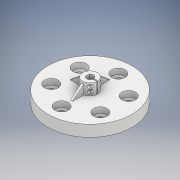
# Autodesk Inventor part: MC001
Saved by Autodesk Inventor 2017 SP1 (Build 210196100, 196)
## iProperties
Created: 2017-06-01
Part Number: MC001
Material: ABS Plastic
Document SubType Name: Modeling
Designer: Zach
Density: 1.06 g/cm^3
Appearance: CR White
Author: Zach
Autodesk Inventor part; units mm, degrees
ref_plane "YZ Plane" through (0, 0, 0) normal (1, 0, 0) x (0, 1, 0)
ref_plane "XY Plane" through (0, 0, 0) normal (0, 0, 1) x (1, 0, 0)
sketch "Sketch1" plane through (0, 0, 0) normal (0, 0, 1) x (1, 0, 0)
  circle A0 centre (0, 0) radius 37
  circle A1 centre (0, 0) radius 3
  circle A2 centre (0, 25) radius 2.575
  circle A3 centre (-21.6506, 12.5) radius 2.575
  circle A4 centre (-21.6506, -12.5) radius 2.575
  circle A5 centre (0, -25) radius 2.575
  circle A6 centre (21.6506, -12.5) radius 2.575
  circle A7 centre (21.6506, 12.5) radius 2.575
  dimension "d0" = 74
  dimension "d1" = 6
  dimension "d2" = 5.15
  dimension "d3" = 25
  dimension "d6" = 360
  constraints: 8 centre point, 2 coincident, 13 other
  measures "d0" diameter of A0
  measures "d1" diameter of A1
  measures "d2" diameter of A2
  measures "d3" distance of point (0, 0) A2.centre
extrude "Extrusion1" add sketch "Sketch1" along normal blind 10
sketch "Sketch2" plane through (0, 0, 10) normal (0, 0, 1) x (1, 0, 0)
  circle A0 centre (0, 0) radius 3 projected
  circle A1 centre (0, 0) radius 6.5
  circle A2 centre (0, 0) radius 3 projected
  dimension "d10" = 13
  constraints: 3 coincident, 1 centre point, 3 other
  measures "d10" diameter of A1
extrude "Extrusion2" add sketch "Sketch2" along normal blind 10
sketch "Sketch3" plane through (0, 0, 10) normal (0, 0, 1) x (1, 0, 0)
  line L0 (0, 0.5) -> (36.9966, 0.5)
  circle A0 centre (0, 0) radius 6.5 projected
  line L1 (0, 0.5) -> (0, -0.5)
  circle A1 centre (0, 0) radius 37 projected
  line L2 (0, -0.5) -> (36.9966, -0.5)
  arc A2 (36.9966, -0.5) -> (36.9966, 0.5) centre (0, 0) ccw
  point P0 (0, 0)
  dimension "d13" = 1
  dimension "d14" = 0.5
  constraints: 6 end point, 4 point on circle, 2 horizontal, 2 vertical alignment, 1 centre point, 1 concentric, 1 midpoint, 1 vertical
  measures "d13" distance of L0.start L1.end
  measures "d14" distance of L0.start point (0, 0)
extrude "Extrusion4" cut sketch "Sketch3" along normal through all contours L0 A0 L2 L1 | L0 A1 L2 A0 picked at (2.1667, 0) picked at (16.6648, -0.2223)
sketch "Sketch4" plane through (0, 0, 0) normal (0, 1, 0) x (-1, 0, 0)
  circle A0 centre (-4.958, 13) radius 1
  circle A1 centre (-4.958, 17) radius 1
  line L0 (-2.958, 10) -> (-6.4807, 10) projected
  line L1 (-6.4807, 20) -> (-2.958, 20) projected
  line L2 (-2.958, 20) -> (-2.958, 10) projected
  point P0 (0, 0)
  dimension "d19" = 2
  dimension "d20" = 2
  dimension "d21" = 3
  dimension "d22" = 3
  dimension "d25" = 2
  dimension "d26" = 2
  constraints: 2 centre point
  measures "d19" diameter of A0
  measures "d20" diameter of A1
  measures "d21" distance from line of A0.centre L0
  measures "d22" distance from line of L1 A1.centre
  measures "d25" distance from line of L2 A0.centre
  measures "d26" distance from line of L2 A1.centre
extrude "Extrusion5" cut sketch "Sketch4" along normal through all both and the other way through all
ref_plane "Work Plane1" through (0, -6.5, 0) normal (0, 1, 0) x (-1, 0, 0)
sketch "Sketch6" plane through (0, -6.5, 0) normal (0, 1, 0) x (-1, 0, 0)
  spline S0 degree 5 poles (-3.958, 13) (-3.958, 13.1746) (-3.9961, 13.3498) (-4.0725, 13.5117) (-4.1803, 13.65) (-4.4348, 13.869) (-4.583, 13.9477) (-4.7351, 13.9925) (-4.882, 14.0068) (-5.1241, 13.9915) (-5.2226, 13.9719) (-5.3158, 13.9412) (-5.403, 13.9006) (-5.5546, 13.8069) (-5.6202, 13.7562) (-5.6812, 13.6984) (-5.7373, 13.6329) (-5.8334, 13.4906) (-5.8743, 13.4151) (-5.9095, 13.3294) (-5.9362, 13.233) (-5.9579, 13.0655) (-5.9613, 13.0002) (-5.9591, 12.9344) (-5.9515, 12.8703) (-5.9066, 12.6381) (-5.84, 12.4944) (-5.7574, 12.3787) (-5.6684, 12.2835) (-5.4331, 12.1055) (-5.2863, 12.0346) (-5.1214, 11.9912) (-4.9425, 11.9823) (-4.6619, 12.04) (-4.5657, 12.0716) (-4.4707, 12.1171) (-4.3797, 12.1768) (-4.1744, 12.3577) (-4.0693, 12.4951) (-3.995, 12.6552) (-3.958, 12.828) (-3.958, 13) knots 0 0 0 0 0 0 0.118573 0.118573 0.118573 0.118573 0.240763 0.240763 0.240763 0.240763 0.331598 0.331598 0.331598 0.331598 0.410987 0.410987 0.410987 0.410987 0.484843 0.484843 0.484843 0.484843 0.529131 0.529131 0.529131 0.529131 0.655639 0.655639 0.655639 0.655639 0.80726 0.80726 0.80726 0.80726 0.884923 0.884923 0.884923 0.884923 1 1 1 1 1 1 projected
  spline S1 degree 5 poles (-3.958, 17) (-3.958, 17.1746) (-3.9961, 17.3498) (-4.0725, 17.5117) (-4.1803, 17.65) (-4.4348, 17.869) (-4.583, 17.9477) (-4.7351, 17.9925) (-4.882, 18.0068) (-5.1241, 17.9915) (-5.2226, 17.9719) (-5.3158, 17.9412) (-5.403, 17.9006) (-5.5546, 17.8069) (-5.6202, 17.7562) (-5.6812, 17.6984) (-5.7373, 17.6329) (-5.8334, 17.4906) (-5.8743, 17.4151) (-5.9095, 17.3294) (-5.9362, 17.233) (-5.9579, 17.0655) (-5.9613, 17.0002) (-5.9591, 16.9344) (-5.9515, 16.8703) (-5.9066, 16.6381) (-5.84, 16.4944) (-5.7574, 16.3787) (-5.6684, 16.2835) (-5.4331, 16.1055) (-5.2863, 16.0346) (-5.1214, 15.9912) (-4.9425, 15.9823) (-4.6619, 16.04) (-4.5657, 16.0716) (-4.4707, 16.1171) (-4.3797, 16.1768) (-4.1744, 16.3577) (-4.0693, 16.4951) (-3.995, 16.6552) (-3.958, 16.828) (-3.958, 17) knots 0 0 0 0 0 0 0.118573 0.118573 0.118573 0.118573 0.240763 0.240763 0.240763 0.240763 0.331598 0.331598 0.331598 0.331598 0.410987 0.410987 0.410987 0.410987 0.484843 0.484843 0.484843 0.484843 0.529131 0.529131 0.529131 0.529131 0.655639 0.655639 0.655639 0.655639 0.80726 0.80726 0.80726 0.80726 0.884923 0.884923 0.884923 0.884923 1 1 1 1 1 1 projected
  circle A0 centre (-4.958, 13) radius 1 projected
  circle A1 centre (-4.958, 17) radius 1 projected
  line L0 (-5.958, 11.2679) -> (-6.958, 13)
  line L1 (-6.958, 13) -> (-5.958, 14.7321)
  line L2 (-5.958, 14.7321) -> (-3.958, 14.7321)
  line L3 (-3.958, 14.7321) -> (-2.958, 13)
  line L4 (-2.958, 13) -> (-3.958, 11.2679)
  line L5 (-3.958, 11.2679) -> (-5.958, 11.2679)
  line L6 (-5.958, 15.2679) -> (-6.958, 17)
  line L7 (-6.958, 17) -> (-5.958, 18.7321)
  line L8 (-5.958, 18.7321) -> (-3.958, 18.7321)
  line L9 (-3.958, 18.7321) -> (-2.958, 17)
  line L10 (-2.958, 17) -> (-3.958, 15.2679)
  line L11 (-3.958, 15.2679) -> (-5.958, 15.2679)
  point P0 (0, 0)
  dimension "d30" = 2
  dimension "d31" = 2
  constraints: 24 end point, 4 horizontal alignment, 2 coincident, 28 other
  measures "d30" distance of L6.end point (-4.958, 17)
  measures "d31" distance of L0.end point (-4.958, 13)
extrude "Extrusion6" cut sketch "Sketch6" along normal blind 3 contours S0 | L0 L1 L2 L3 L4 L5 | L6 L7 L8 L9 L10 L11
sketch "Sketch7" plane through (0, 0, 0) normal (1, 0, 0) x (0, 1, 0)
  line L0 (6.5, 18) -> (16.5, 10)
  line L1 (37, 10) -> (-37, 10) projected
  line L2 (-6.5, 10) -> (6.5, 10) projected
  line L3 (6.5, 10) -> (16.5, 10)
  line L4 (6.5, 10) -> (5.5, 10)
  line L5 (5.5, 10) -> (5.5, 18)
  line L6 (5.5, 18) -> (6.5, 18)
  line L7 (6.5, 10) -> (6.5, 20) projected
  line L8 (0, 0) -> (0, 35.1607) construction
  line L9 (-6.5, 18) -> (-16.5, 10)
  line L10 (-37, 10) -> (37, 10)
  line L11 (6.5, 10) -> (-6.5, 10)
  line L12 (-6.5, 10) -> (-16.5, 10)
  line L13 (-6.5, 10) -> (-5.5, 10)
  line L14 (-5.5, 10) -> (-5.5, 18)
  line L15 (-5.5, 18) -> (-6.5, 18)
  point P0 (-0.5, 10)
  point P1 (0.5, 10)
  dimension "d36" = 10
  dimension "d39" = 8
  dimension "d46" = 1
  dimension "d53" = 10
  constraints: 26 end point, 7 symmetric about line, 5 point on line, 2 vertical, 1 perpendicular, 2 other
  measures "d36" horizontal distance of L0.start L0.end
  measures "d39" vertical distance of L0.start L0.end
  measures "d46" distance of L2.end L4.end
  measures "d53" horizontal distance of L9.start L9.end
extrude "Extrusion7" add sketch "Sketch7" along normal mid plane 2
sketch "Sketch8" plane through (0, 0, 0) normal (0, 1, 0) x (-1, 0, 0)
  line L0 (6.5, 18) -> (16.5, 10)
  line L1 (37, 10) -> (-37, 10) projected
  line L2 (3.7682, 10) -> (3.7682, 20.1855)
  line L3 (16.5, 10) -> (3.7682, 10)
  line L4 (6.5, 18) -> (5.5, 18)
  line L5 (6.5, 10) -> (6.5, 20) projected
  line L6 (6.5, 18) -> (7.5, 18) construction
  line L7 (5.5, 18) -> (5.5, 10)
  line L8 (1, 10) -> (6.5, 10) projected
  line L9 (6.5, 10) -> (5.5, 10)
  point P0 (0, 0)
  dimension "d42" = 10
  dimension "d43" = 8
  dimension "d51" = 1
  dimension "d52" = 180
  constraints: 14 end point, 4 point on line, 2 collinear, 2 perpendicular, 2 vertical, 1 horizontal
  measures "d42" horizontal distance of L0.start L0.end
  measures "d43" vertical distance of L0.start L0.end
  measures "d51" distance of L0.start L4.end
  measures "d52" angle of L4 L6
extrude "Extrusion8" add sketch "Sketch8" along normal mid plane 2
sketch "Sketch9" plane through (0, 0, 0) normal (0, 0, -1) x (-1, 0, 0)
  circle A0 centre (0, 0) radius 3 projected
  line L0 (2.5, -1.6583) -> (2.5, 1.6583)
  arc A1 (2.5, -1.6583) -> (2.5, 1.6583) centre (0, 0) ccw
  dimension "d54" = 2.5
  constraints: 4 point on circle, 2 end point, 1 centre point, 1 concentric, 1 vertical
  measures "d54" distance from line of point (0, 0) L0
extrude "Extrusion9" add sketch "Sketch9" against normal blind 20 contours A0 L0 picked at (2.5914, -0.3806)
sketch "Sketch10" plane through (0, 0, 10) normal (0, 0, 1) x (1, 0, 0)
  circle A0 centre (0, 0) radius 37 projected
  line L0 (-6.4226, -1) -> (-16.5, -1) projected
  line L1 (-16.5, -1) -> (-16.5, 1) projected
  line L2 (-16.5, 1) -> (-6.4226, 1) projected
  arc A1 (-1, 6.4226) -> (-6.4226, 1) centre (0, 0) ccw projected
  line L3 (-1, 6.4226) -> (-1, 16.5) projected
  line L4 (-1, 16.5) -> (1, 16.5) projected
  line L5 (1, 16.5) -> (1, 6.4226) projected
  arc A2 (6.4807, 0.5) -> (1, 6.4226) centre (0, 0) ccw projected
  line L6 (6.4807, 0.5) -> (2.958, 0.5) projected
  arc A3 (2.958, -0.5) -> (2.958, 0.5) centre (0, 0) ccw projected
  line L7 (2.958, -0.5) -> (6.4807, -0.5) projected
  arc A4 (1, -6.4226) -> (6.4807, -0.5) centre (0, 0) ccw projected
  line L8 (1, -6.4226) -> (1, -16.5) projected
  line L9 (1, -16.5) -> (-1, -16.5) projected
  line L10 (-1, -16.5) -> (-1, -6.4226) projected
  arc A5 (-6.4226, -1) -> (-1, -6.4226) centre (0, 0) ccw projected
  circle A6 centre (21.6506, 12.5) radius 2.575 projected
  circle A7 centre (21.6506, -12.5) radius 2.575 projected
  circle A8 centre (0, -25) radius 2.575 projected
  circle A9 centre (-21.6506, -12.5) radius 2.575 projected
  circle A10 centre (-21.6506, 12.5) radius 2.575 projected
  circle A11 centre (0, 25) radius 2.575 projected
  circle A12 centre (0, 25) radius 6
  circle A13 centre (-21.6506, 12.5) radius 6
  circle A14 centre (-21.6506, -12.5) radius 6
  circle A15 centre (0, -25) radius 6
  circle A16 centre (21.6506, -12.5) radius 6
  circle A17 centre (21.6506, 12.5) radius 6
  dimension "d57" = 12
  dimension "d60" = 360
  constraints: 6 centre point, 6 coincident, 19 other
  measures "d57" diameter of A12
extrude "Extrusion10" cut sketch "Sketch10" against normal blind 5 contours A12 | A13 | A14 | A15 | A16 | A17
body "Solid1"
